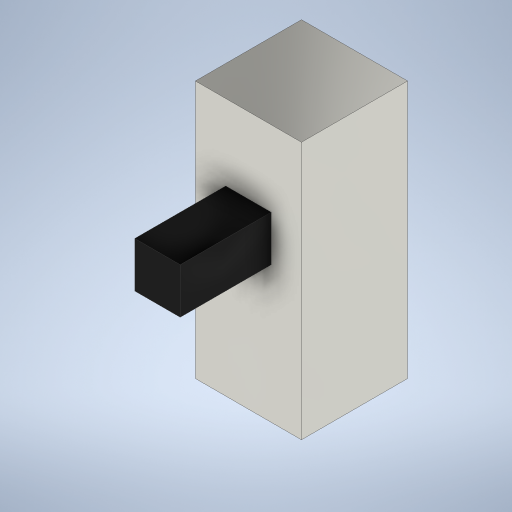
# Autodesk Inventor part: Switch
Saved by Autodesk Inventor 2024.3 (Build 283343000, 343)
## iProperties
Created: 2025-01-23
Part Number: Switch
Material: Generic
Document SubType Name: Modeling
Designer: ASUS TUF
Density: 1 g/cm^3
Appearance: Default
Author: ASUS TUF
Autodesk Inventor part; units mm, degrees
ref_plane "YZ Plane" through (0, 0, 0) normal (1, 0, 0) x (0, 1, 0)
ref_plane "XZ Plane" through (0, 0, 0) normal (0, 1, 0) x (-1, 0, 0)
ref_plane "XY Plane" through (0, 0, 0) normal (0, 0, 1) x (1, 0, 0)
sketch "Sketch1" plane through (0, 0, 0) normal (0, 0, 1) x (1, 0, 0)
  line L0 (-1.75, -4.25) -> (1.75, -4.25)
  line L1 (1.75, -4.25) -> (1.75, 4.25)
  line L2 (1.75, 4.25) -> (-1.75, 4.25)
  line L3 (-1.75, 4.25) -> (-1.75, -4.25)
  line L4 (-1.75, -4.25) -> (1.75, 4.25) construction
  line L5 (1.75, -4.25) -> (-1.75, 4.25) construction
  point P0 (0, 0)
  dimension "d0" = 3.5
  dimension "d1" = 8.5
  constraints: 12 end point, 2 midpoint, 2 parallel, 1 horizontal, 1 perpendicular
  measures "d0" distance of L2.end L1.end
  measures "d1" distance of L1.end L0.end
extrude "Extrusion1" add sketch "Sketch1" along normal blind 3.5
sketch "Sketch2" plane through (0, 0, 3.5) normal (0, 0, 1) x (1, 0, 0)
  line L0 (-0.75, 0.25) -> (0.75, 0.25)
  line L1 (0.75, 0.25) -> (0.75, 1.75)
  line L2 (0.75, 1.75) -> (-0.75, 1.75)
  line L3 (-0.75, 1.75) -> (-0.75, 0.25)
  line L4 (-0.75, 0.25) -> (0.75, 1.75) construction
  line L5 (0.75, 0.25) -> (-0.75, 1.75) construction
  line L6 (1.75, 4.25) -> (-1.75, 4.25) projected
  point P0 (0, 0)
  point P1 (0, 1)
  dimension "d4" = 1.5
  dimension "d5" = 1.5
  dimension "d6" = 4
  constraints: 12 end point, 2 midpoint, 2 parallel, 1 horizontal, 1 perpendicular, 1 vertical alignment
  measures "d4" distance of L2.end L1.end
  measures "d5" distance of L1.end L0.end
  measures "d6" distance between parallel lines of L6 L0
extrude "Extrusion2" add sketch "Sketch2" along normal blind 3
body "Solid1"
